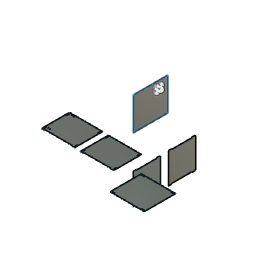
Optical Path Casing (Autodesk Fusion 360 design; units mm, degrees)
Autodesk Fusion 360 part; units mm, degrees
sketch "Sketch2" plane through (0, 0, 0) normal (0, 0, 1) x (1, 0, 0)
  line L0 (32.2949, 19.5332) -> (252.2949, 19.5332)
  line L1 (252.2949, 19.5332) -> (252.2949, -180.4668)
  line L2 (252.2949, -180.4668) -> (32.2949, -180.4668)
  line L3 (32.2949, -180.4668) -> (32.2949, 19.5332)
  line L4 (35.7949, 16.0332) -> (56.7949, 16.0332)
  line L5 (56.7949, 16.0332) -> (56.7949, 12.3332)
  line L6 (56.7949, 12.3332) -> (35.7949, 12.3332)
  line L7 (35.7949, 12.3332) -> (35.7949, 16.0332)
  line L8 (35.7949, -173.2668) -> (56.7949, -173.2668)
  line L9 (56.7949, -173.2668) -> (56.7949, -176.9668)
  line L10 (56.7949, -176.9668) -> (35.7949, -176.9668)
  line L11 (35.7949, -176.9668) -> (35.7949, -173.2668)
  line L12 (227.7949, -173.2668) -> (248.7949, -173.2668)
  line L13 (248.7949, -173.2668) -> (248.7949, -176.9668)
  line L14 (248.7949, -176.9668) -> (227.7949, -176.9668)
  line L15 (227.7949, -176.9668) -> (227.7949, -173.2668)
  line L16 (227.7949, 16.0332) -> (248.7949, 16.0332)
  line L17 (248.7949, 16.0332) -> (248.7949, 12.3332)
  line L18 (248.7949, 12.3332) -> (227.7949, 12.3332)
  line L19 (227.7949, 12.3332) -> (227.7949, 16.0332)
  dimension "d3" = 220
  dimension "d4" = 200
  dimension "d5" = 21
  dimension "d6" = 3.7
  dimension "d7" = 3.5
  dimension "d8" = 3.5
  dimension "d9" = 21
  dimension "d10" = 3.7
  dimension "d11" = 3.5
  dimension "d12" = 3.5
  dimension "d13" = 21
  dimension "d14" = 3.7
  dimension "d15" = 3.5
  dimension "d16" = 3.5
  dimension "d17" = 21
  dimension "d18" = 3.7
  dimension "d19" = 3.5
  dimension "d20" = 3.5
  constraint horizontal L0
  constraint vertical L1
  constraint horizontal L2
  constraint vertical L3
  constraint horizontal L4
  constraint vertical L5
  constraint horizontal L6
  constraint vertical L7
  constraint horizontal L8
  constraint vertical L9
  constraint horizontal L10
  constraint vertical L11
  constraint horizontal L12
  constraint vertical L13
  constraint horizontal L14
  constraint vertical L15
  constraint horizontal L16
  constraint vertical L17
  constraint horizontal L18
  constraint vertical L19
  measures "d3" distance of L0.start L0.end
  measures "d4" distance of L0.start L2.end
  measures "d5" distance of L4.start L4.end
  measures "d6" distance of L4.start L6.end
  measures "d7" distance of L0 L4
  measures "d8" distance of L3 L7
  measures "d9" distance of L8.start L8.end
  measures "d10" distance of L8.start L10.end
  measures "d11" distance of L3 L11
  measures "d12" distance of L2 L10
  measures "d13" distance of L12.start L12.end
  measures "d14" distance of L12.start L14.end
  measures "d15" distance of L2 L14
  measures "d16" distance of L1 L13
  measures "d17" distance of L16.start L16.end
  measures "d18" distance of L16.start L18.end
  measures "d19" distance of L0 L16
  measures "d20" distance of L1 L16.end
sketch "Sketch3" plane through (0, 0, 0) normal (1, 0, 0) x (0, 1, 0)
  line L0 (-1, 5) -> (174, 5)
  line L1 (174, 5) -> (174, -184.5)
  line L2 (174, -184.5) -> (-1, -184.5)
  line L3 (-1, -184.5) -> (-1, 5)
  line L4 (19, 5.0067) -> (-1, 5.0067)
  line L5 (-1, -184.5) -> (19, -184.5)
  line L6 (19, -184.5) -> (19, -188.5)
  line L7 (19, -188.5) -> (-1, -188.5)
  line L8 (-1, -188.5) -> (-1, -184.5)
  line L9 (174, -184.5) -> (164, -184.5)
  line L10 (174, 5) -> (164, 5)
  line L11 (34, -147.5) -> (19, -147.5)
  line L12 (19, -147.5) -> (19, -167.5)
  line L13 (19, -167.5) -> (34, -167.5)
  line L14 (34, -167.5) -> (34, -147.5)
  line L15 (170.5, -184.5) -> (150.5, -184.5)
  line L16 (150.5, -184.5) -> (150.5, -188.5)
  line L17 (150.5, -188.5) -> (170.5, -188.5)
  line L18 (170.5, -188.5) -> (170.5, -184.5)
  line L19 (170.5, 5) -> (150.5, 5)
  line L20 (150.5, 5) -> (150.5, 9)
  line L21 (150.5, 9) -> (170.5, 9)
  line L22 (170.5, 9) -> (170.5, 5)
  line L23 (377.0199, -182.529) -> (377.0199, -186.529)
  line L24 (400.5199, 6.971) -> (400.5199, -182.529)
  line L25 (397.0199, -182.529) -> (377.0199, -182.529)
  line L26 (397.0199, 10.971) -> (397.0199, 6.971)
  line L27 (225.5199, -182.529) -> (225.5199, 6.971)
  line L28 (400.5199, -182.529) -> (380.5199, -182.529)
  line L29 (245.5199, -186.529) -> (225.5199, -186.529)
  line L30 (225.5199, -182.529) -> (245.5199, -182.529)
  line L31 (377.0199, 10.971) -> (397.0199, 10.971)
  line L32 (225.5199, 6.971) -> (400.5199, 6.971)
  line L33 (397.0199, -186.529) -> (397.0199, -182.529)
  line L34 (400.5199, -182.529) -> (225.5199, -182.529)
  line L35 (377.0199, 6.971) -> (377.0199, 10.971)
  line L36 (377.0199, -186.529) -> (397.0199, -186.529)
  line L37 (397.0199, 6.971) -> (377.0199, 6.971)
  line L38 (400.5199, 6.971) -> (380.5199, 6.971)
  line L39 (225.5199, -186.529) -> (225.5199, -182.529)
  line L40 (245.5199, -182.529) -> (245.5199, -186.529)
  line L41 (-1, 5) -> (19, 5)
  line L42 (19, 5) -> (19, 9)
  line L43 (19, 9) -> (-1, 9)
  line L44 (-1, 9) -> (-1, 5)
  line L45 (225.5199, 6.971) -> (245.5199, 6.971)
  line L46 (225.5199, 6.971) -> (245.5199, 6.971)
  line L47 (245.5199, 6.971) -> (245.5199, 10.971)
  line L48 (245.5199, 10.971) -> (225.5199, 10.971)
  line L49 (225.5199, 10.971) -> (225.5199, 6.971)
  point P0 (216.5199, 1.971)
  dimension "d29" = 189.5
  dimension "d30" = 175
  dimension "d33" = 20
  dimension "d34" = 4
  dimension "d39" = 15
  dimension "d40" = 20
  dimension "d41" = 20
  dimension "d42" = 17
  dimension "d103" = 20
  dimension "d104" = 4
  dimension "d105" = 3.5
  dimension "d106" = 20
  dimension "d107" = 4
  dimension "d108" = 3.5
  dimension "d109" = 189.5
  dimension "d110" = 175
  dimension "d113" = 20
  dimension "d114" = 4
  dimension "d119" = 20
  dimension "d120" = 4
  dimension "d121" = 3.5
  dimension "d122" = 20
  dimension "d123" = 4
  dimension "d124" = 3.5
  dimension "d163" = 20
  dimension "d164" = 4
  dimension "d167" = 20
  dimension "d169" = 20
  dimension "d170" = 4
  constraint horizontal L0
  constraint vertical L1
  constraint horizontal L2
  constraint vertical L3
  constraint horizontal L4
  constraint horizontal L5
  constraint vertical L6
  constraint horizontal L7
  constraint vertical L8
  constraint horizontal L9
  constraint horizontal L10
  constraint horizontal L11
  constraint vertical L12
  constraint horizontal L13
  constraint vertical L14
  constraint horizontal L15
  constraint vertical L16
  constraint horizontal L17
  constraint vertical L18
  constraint coincident L2 L15.start
  constraint horizontal L19
  constraint vertical L20
  constraint horizontal L21
  constraint vertical L22
  constraint coincident L10 L19.start
  constraint horizontal L32
  constraint vertical L24
  constraint horizontal L34
  constraint vertical L27
  constraint horizontal L30
  constraint vertical L40
  constraint horizontal L29
  constraint vertical L39
  constraint horizontal L28
  constraint horizontal L38
  constraint horizontal L25
  constraint vertical L23
  constraint horizontal L36
  constraint vertical L33
  constraint coincident L25.start L34
  constraint horizontal L37
  constraint vertical L35
  constraint horizontal L31
  constraint vertical L26
  constraint coincident L26.end L38
  constraint horizontal L41
  constraint vertical L42
  constraint horizontal L43
  constraint vertical L44
  constraint horizontal L45
  constraint horizontal L46
  constraint vertical L47
  constraint horizontal L48
  constraint vertical L49
  measures "d29" distance of L0.start L2.end
  measures "d30" distance of L0.start L0.end
  measures "d33" distance of L2.end L5.end
  measures "d34" distance of L2.end L7.end
  measures "d39" distance of L11.start L11.end
  measures "d40" distance of L11.start L13.end
  measures "d41" distance of L3 L12
  measures "d42" distance of L2 L13
  measures "d103" distance of L15.start L15.end
  measures "d104" distance of L15.start L17.end
  measures "d105" distance of L1 L18
  measures "d106" distance of L19.start L19.end
  measures "d107" distance of L19.start L21.end
  measures "d108" distance of L1 L22
  measures "d109" distance of L27.start L27.end
  measures "d110" distance of L24.start L27.end
  measures "d113" distance of L27.start L30.end
  measures "d114" distance of L27.start L29.end
  measures "d119" distance of L25.start L23.start
  measures "d120" distance of L25.start L33.start
  measures "d121" distance of L24 L33
  measures "d122" distance of L35.start L26.end
  measures "d123" distance of L26.start L26.end
  measures "d124" distance of L24 L26
  measures "d163" distance of L0.start L41.end
  measures "d164" distance of L0.start L43.end
  measures "d167" distance of L27.end L45.end
  measures "d169" distance of L27.end L45.end
  measures "d170" distance of L27.end L48.end
sketch "Sketch5" plane through (0, 0, 0) normal (0, 0, 1) x (1, 0, 0)
  line L0 (-287.8095, 127.6155) -> (-74.8095, 127.6155)
  line L1 (-74.8095, 127.6155) -> (-74.8095, -47.3845)
  line L2 (-74.8095, -47.3845) -> (-287.8095, -47.3845)
  line L3 (-287.8095, -47.3845) -> (-287.8095, 127.6155)
  line L4 (-287.8095, -47.3845) -> (-267.8095, -47.3845)
  line L5 (-267.8095, -47.3845) -> (-267.8095, -50.8845)
  line L6 (-267.8095, -50.8845) -> (-287.8095, -50.8845)
  line L7 (-287.8095, -50.8845) -> (-287.8095, -47.3845)
  line L8 (-74.8095, -47.3845) -> (-94.8095, -47.3845)
  line L9 (-94.8095, -47.3845) -> (-94.8095, -50.8845)
  line L10 (-94.8095, -50.8845) -> (-74.8095, -50.8845)
  line L11 (-74.8095, -50.8845) -> (-74.8095, -47.3845)
  line L12 (-284.3095, -47.3835) -> (-280.6095, -47.3835)
  line L13 (-280.6095, -47.3835) -> (-280.6095, -26.3835)
  line L14 (-280.6095, -26.3835) -> (-284.3095, -26.3835)
  line L15 (-284.3095, -26.3835) -> (-284.3095, -47.3835)
  line L16 (-78.3095, -47.3348) -> (-82.0095, -47.3348)
  line L17 (-82.0095, -47.3348) -> (-82.0095, -26.3348)
  line L18 (-82.0095, -26.3348) -> (-78.3095, -26.3348)
  line L19 (-78.3095, -26.3348) -> (-78.3095, -47.3348)
  line L20 (-326.8625, -44.8366) -> (-539.8625, -44.8366)
  line L21 (-326.8625, -44.8366) -> (-346.8625, -44.8366)
  line L22 (-330.3625, -44.7869) -> (-334.0625, -44.7869)
  line L23 (-326.8625, -48.3366) -> (-326.8625, -44.8366)
  line L24 (-539.8625, 130.1634) -> (-326.8625, 130.1634)
  line L25 (-330.3625, -23.7869) -> (-330.3625, -44.7869)
  line L26 (-346.8625, -48.3366) -> (-326.8625, -48.3366)
  line L27 (-334.0625, -44.7869) -> (-334.0625, -23.7869)
  line L28 (-346.8625, -44.8366) -> (-346.8625, -48.3366)
  line L29 (-334.0625, -23.7869) -> (-330.3625, -23.7869)
  line L30 (-532.6625, -23.8356) -> (-536.3625, -23.8356)
  line L31 (-539.8625, -48.3366) -> (-539.8625, -44.8366)
  line L32 (-536.3625, -44.8356) -> (-532.6625, -44.8356)
  line L33 (-519.8625, -48.3366) -> (-539.8625, -48.3366)
  line L34 (-539.8625, -44.8366) -> (-539.8625, 130.1634)
  line L35 (-519.8625, -44.8366) -> (-519.8625, -48.3366)
  line L36 (-326.8625, 130.1634) -> (-326.8625, -44.8366)
  line L37 (-536.3625, -23.8356) -> (-536.3625, -44.8356)
  line L38 (-532.6625, -44.8356) -> (-532.6625, -23.8356)
  line L39 (-539.8625, -44.8366) -> (-519.8625, -44.8366)
  circle A0 centre (-521, -24.8366) radius 2
  circle A1 centre (-510, -24.8366) radius 2
  line L40 (-536.3625, 126.6634) -> (-532.6625, 126.6634)
  line L41 (-532.6625, 126.6634) -> (-532.6625, 105.6634)
  line L42 (-532.6625, 105.6634) -> (-536.3625, 105.6634)
  line L43 (-536.3625, 105.6634) -> (-536.3625, 126.6634)
  line L44 (-334.0625, 126.6634) -> (-330.3625, 126.6634)
  line L45 (-330.3625, 126.6634) -> (-330.3625, 105.6634)
  line L46 (-330.3625, 105.6634) -> (-334.0625, 105.6634)
  line L47 (-334.0625, 105.6634) -> (-334.0625, 126.6634)
  line L48 (-284.3095, 124.1155) -> (-280.6095, 124.1155)
  line L49 (-280.6095, 124.1155) -> (-280.6095, 103.1155)
  line L50 (-280.6095, 103.1155) -> (-284.3095, 103.1155)
  line L51 (-284.3095, 103.1155) -> (-284.3095, 124.1155)
  line L52 (-82.0095, 124.1155) -> (-78.3095, 124.1155)
  line L53 (-78.3095, 124.1155) -> (-78.3095, 103.1155)
  line L54 (-78.3095, 103.1155) -> (-82.0095, 103.1155)
  line L55 (-82.0095, 103.1155) -> (-82.0095, 124.1155)
  line L56 (-497.8625, 124.1634) -> (-519.8625, 124.1634)
  line L57 (-519.8625, 124.1634) -> (-519.8625, 121.1634)
  line L58 (-519.8625, 121.1634) -> (-497.8625, 121.1634)
  line L59 (-497.8625, 121.1634) -> (-497.8625, 124.1634)
  dimension "d57" = 213
  dimension "d58" = 175
  dimension "d59" = 20
  dimension "d60" = 3.5
  dimension "d61" = 20
  dimension "d62" = 3.5
  dimension "d63" = 3.7
  dimension "d64" = 21
  dimension "d65" = 0.001
  dimension "d66" = 3.5
  dimension "d67" = 3.7
  dimension "d68" = 21
  dimension "d69" = 3.5
  dimension "d70" = 213
  dimension "d71" = 175
  dimension "d72" = 20
  dimension "d73" = 3.5
  dimension "d74" = 20
  dimension "d75" = 3.5
  dimension "d76" = 3.7
  dimension "d77" = 21
  dimension "d78" = 0.001
  dimension "d79" = 3.5
  dimension "d80" = 3.7
  dimension "d81" = 21
  dimension "d82" = 3.5
  dimension "d83" = 4
  dimension "d84" = 4
  dimension "d85" = 11
  dimension "d86" = 20
  dimension "d87" = 3.7
  dimension "d88" = 21
  dimension "d89" = 3.5
  dimension "d90" = 3.5
  dimension "d91" = 3.7
  dimension "d92" = 21
  dimension "d93" = 3.5
  dimension "d94" = 3.5
  dimension "d95" = 3.7
  dimension "d96" = 21
  dimension "d97" = 3.5
  dimension "d98" = 3.5
  dimension "d99" = 3.7
  dimension "d100" = 21
  dimension "d101" = 3.5
  dimension "d102" = 3.5
  dimension "d125" = 22
  dimension "d126" = 3
  dimension "d127" = 6
  dimension "d128" = 20
  constraint horizontal L0
  constraint vertical L1
  constraint horizontal L2
  constraint vertical L3
  constraint horizontal L4
  constraint vertical L5
  constraint horizontal L6
  constraint vertical L7
  constraint horizontal L8
  constraint vertical L9
  constraint horizontal L10
  constraint vertical L11
  constraint horizontal L12
  constraint vertical L13
  constraint horizontal L14
  constraint vertical L15
  constraint horizontal L16
  constraint vertical L17
  constraint horizontal L18
  constraint vertical L19
  constraint horizontal L24
  constraint vertical L36
  constraint horizontal L20
  constraint vertical L34
  constraint horizontal L39
  constraint vertical L35
  constraint horizontal L33
  constraint vertical L31
  constraint horizontal L21
  constraint vertical L28
  constraint horizontal L26
  constraint vertical L23
  constraint horizontal L32
  constraint vertical L38
  constraint horizontal L30
  constraint vertical L37
  constraint horizontal L22
  constraint vertical L27
  constraint horizontal L29
  constraint vertical L25
  constraint horizontal L40
  constraint vertical L41
  constraint horizontal L42
  constraint vertical L43
  constraint horizontal L44
  constraint vertical L45
  constraint horizontal L46
  constraint vertical L47
  constraint horizontal L48
  constraint vertical L49
  constraint horizontal L50
  constraint vertical L51
  constraint horizontal L52
  constraint vertical L53
  constraint horizontal L54
  constraint vertical L55
  constraint horizontal L56
  constraint vertical L57
  constraint horizontal L58
  constraint vertical L59
  measures "d57" distance of L0.start L0.end
  measures "d58" distance of L0.start L2.end
  measures "d59" distance of L2.end L4.end
  measures "d60" distance of L2.end L6.end
  measures "d61" distance of L1.end L8.end
  measures "d62" distance of L1.end L10.end
  measures "d63" distance of L12.start L12.end
  measures "d64" distance of L12.start L14.end
  measures "d65" distance of L2 L12
  measures "d66" distance of L3 L15
  measures "d67" distance of L16.start L16.end
  measures "d68" distance of L16.start L18.end
  measures "d69" distance of L1 L19
  measures "d70" distance of L24.end L24.start
  measures "d71" distance of L20.end L24.start
  measures "d72" distance of L20.end L35.start
  measures "d73" distance of L20.end L31.start
  measures "d74" distance of L20.start L21.end
  measures "d75" distance of L20.start L23.start
  measures "d76" distance of L32.start L32.end
  measures "d77" distance of L32.start L30.end
  measures "d78" distance of L20 L32
  measures "d79" distance of L34 L37
  measures "d80" distance of L22.end L22.start
  measures "d81" distance of L22.start L25.start
  measures "d82" distance of L25 L36
  measures "d83" diameter of A0
  measures "d84" diameter of A1
  measures "d85" distance of A0.centre A1.centre
  measures "d86" distance of L20 A0.centre
  measures "d87" distance of L40.start L40.end
  measures "d88" distance of L40.start L42.end
  measures "d89" distance of L34 L43
  measures "d90" distance of L24 L40
  measures "d91" distance of L44.start L44.end
  measures "d92" distance of L44.start L46.end
  measures "d93" distance of L36 L45
  measures "d94" distance of L24 L44.start
  measures "d95" distance of L48.start L48.end
  measures "d96" distance of L48.start L50.end
  measures "d97" distance of L0 L48
  measures "d98" distance of L3 L51
  measures "d99" distance of L52.start L52.end
  measures "d100" distance of L52.start L54.end
  measures "d101" distance of L1 L53
  measures "d102" distance of L0 L52
  measures "d125" distance of L56.start L56.end
  measures "d126" distance of L56 L58
  measures "d127" distance of L24 L56
  measures "d128" distance of L34 L57
extrude "Extrude1" add sketch "Sketch5" along normal blind 1 contours L20 L21 L24 L34 L36 L39 makes body 1
extrude "Extrude2" add sketch "Sketch5" along normal blind 1 contours L20 L31 L33 L35 L39 bodies 1
extrude "Extrude3" add sketch "Sketch5" along normal blind 1 contours L20 L21 L23 L26 L28 bodies 1
extrude "Extrude4" add sketch "Sketch5" along normal blind 1 separate body contours L0 L1 L2 L3 L4 L8 makes body 2
extrude "Extrude5" add sketch "Sketch5" along normal blind 1 contours L2 L4 L5 L6 L7 bodies 2
extrude "Extrude6" add sketch "Sketch5" along normal blind 1 contours L2 L8 L9 L10 L11 bodies 2
extrude "Extrude7" add sketch "Sketch2" along normal blind 1 separate body makes body 3
extrude "Extrude8" add sketch "Sketch3" along normal blind 1 separate body contours L24 L25 L27 L28 L30 L32 L34 L37 L38 L45 L46 makes body 4
extrude "Extrude9" add sketch "Sketch3" along normal blind 1 contours L29 L30 L34 L39 L40 bodies 4
extrude "Extrude10" add sketch "Sketch3" along normal blind 1 contours L23 L25 L28 L33 L34 L36 bodies 4
extrude "Extrude11" add sketch "Sketch3" along normal blind 1 separate body contours L0 L1 L2 L3 L5 L9 L10 L15 L19 L41 makes body 5
extrude "Extrude12" add sketch "Sketch3" along normal blind 1 contours L2 L9 L15 L16 L17 L18 bodies 5
extrude "Extrude13" add sketch "Sketch3" along normal blind 1 contours L2 L5 L6 L7 L8 bodies 5
extrude "Extrude14" add sketch "Sketch3" along normal blind 1 separate body contours L0 L4 L41 L42 L44 | L4 L42 L43 L44 makes body 6
extrude "Extrude15" add sketch "Sketch3" along normal blind 1 contours L0 L10 L19 L20 L21 L22 bodies 5
extrude "Extrude17" add sketch "Sketch3" along normal blind 1 contours L26 L31 L32 L35 L37 L38 bodies 4
combine "Combine1" operation add target body 5 tool bodies 6
extrude "Extrude18" add sketch "Sketch3" along normal blind 1 contours L32 L45 L46 L47 L48 L49 bodies 4
sketch "Side 2" plane through (0, 0, 1) normal (0, 0, 1) x (-1, 0, 0)
  line L0 (497.8625, -124.1634) -> (497.8625, -121.1634)
  line L1 (497.8625, -121.1634) -> (519.8625, -121.1634)
  line L2 (519.8625, -121.1634) -> (519.8625, -124.1634)
  line L3 (519.8625, -124.1634) -> (497.8625, -124.1634)
  line L4 (330.3625, -105.6634) -> (334.0625, -105.6634)
  line L5 (334.0625, -105.6634) -> (334.0625, -126.6634)
  line L6 (334.0625, -126.6634) -> (330.3625, -126.6634)
  line L7 (330.3625, -126.6634) -> (330.3625, -105.6634)
  circle A0 centre (521, 24.8366) radius 2
  circle A1 centre (510, 24.8366) radius 2
  line L8 (532.6625, -105.6634) -> (536.3625, -105.6634)
  line L9 (536.3625, -105.6634) -> (536.3625, -126.6634)
  line L10 (536.3625, -126.6634) -> (532.6625, -126.6634)
  line L11 (532.6625, -126.6634) -> (532.6625, -105.6634)
  line L12 (532.6625, 23.8356) -> (532.6625, 44.8356)
  line L13 (532.6625, 44.8356) -> (536.3625, 44.8356)
  line L14 (536.3625, 44.8356) -> (536.3625, 23.8356)
  line L15 (536.3625, 23.8356) -> (532.6625, 23.8356)
  line L16 (334.0625, 44.7869) -> (334.0625, 23.7869)
  line L17 (334.0625, 23.7869) -> (330.3625, 23.7869)
  line L18 (330.3625, 23.7869) -> (330.3625, 44.7869)
  line L19 (330.3625, 44.7869) -> (334.0625, 44.7869)
  line L20 (539.8625, -130.1634) -> (539.8625, 48.3366)
  line L21 (539.8625, 48.3366) -> (519.8625, 48.3366)
  line L22 (519.8625, 48.3366) -> (519.8625, 44.8366)
  line L23 (519.8625, 44.8366) -> (346.8625, 44.8366)
  line L24 (346.8625, 44.8366) -> (346.8625, 48.3366)
  line L25 (346.8625, 48.3366) -> (326.8625, 48.3366)
  line L26 (326.8625, 48.3366) -> (326.8625, -130.1634)
  line L27 (326.8625, -130.1634) -> (539.8625, -130.1634)
sketch "Side 3" plane through (0, 0, 1) normal (0, 0, 1) x (-1, 0, 0)
  line L0 (280.6095, -103.1155) -> (284.3095, -103.1155)
  line L1 (284.3095, -103.1155) -> (284.3095, -124.1155)
  line L2 (284.3095, -124.1155) -> (280.6095, -124.1155)
  line L3 (280.6095, -124.1155) -> (280.6095, -103.1155)
  line L4 (78.3095, -103.1155) -> (82.0095, -103.1155)
  line L5 (82.0095, -103.1155) -> (82.0095, -124.1155)
  line L6 (82.0095, -124.1155) -> (78.3095, -124.1155)
  line L7 (78.3095, -124.1155) -> (78.3095, -103.1155)
  line L8 (284.3095, 47.3835) -> (284.3095, 26.3835)
  line L9 (284.3095, 26.3835) -> (280.6095, 26.3835)
  line L10 (280.6095, 26.3835) -> (280.6095, 47.3835)
  line L11 (280.6095, 47.3835) -> (284.3095, 47.3835)
  line L12 (82.0095, 26.3348) -> (78.3095, 26.3348)
  line L13 (78.3095, 26.3348) -> (78.3095, 47.3348)
  line L14 (78.3095, 47.3348) -> (82.0095, 47.3348)
  line L15 (82.0095, 47.3348) -> (82.0095, 26.3348)
  line L16 (267.8095, 47.3845) -> (94.8095, 47.3845)
  line L17 (94.8095, 47.3845) -> (94.8095, 50.8845)
  line L18 (94.8095, 50.8845) -> (74.8095, 50.8845)
  line L19 (74.8095, 50.8845) -> (74.8095, -127.6155)
  line L20 (74.8095, -127.6155) -> (287.8095, -127.6155)
  line L21 (287.8095, -127.6155) -> (287.8095, 50.8845)
  line L22 (287.8095, 50.8845) -> (267.8095, 50.8845)
  line L23 (267.8095, 50.8845) -> (267.8095, 47.3845)
sketch "Bottom" plane through (0, 0, 1) normal (0, 0, 1) x (-1, 0, 0)
  line L0 (-56.7949, 176.9668) -> (-35.7949, 176.9668)
  line L1 (-35.7949, 176.9668) -> (-35.7949, 173.2668)
  line L2 (-35.7949, 173.2668) -> (-56.7949, 173.2668)
  line L3 (-56.7949, 173.2668) -> (-56.7949, 176.9668)
  line L4 (-248.7949, 176.9668) -> (-227.7949, 176.9668)
  line L5 (-227.7949, 176.9668) -> (-227.7949, 173.2668)
  line L6 (-227.7949, 173.2668) -> (-248.7949, 173.2668)
  line L7 (-248.7949, 173.2668) -> (-248.7949, 176.9668)
  line L8 (-248.7949, -12.3332) -> (-227.7949, -12.3332)
  line L9 (-227.7949, -12.3332) -> (-227.7949, -16.0332)
  line L10 (-227.7949, -16.0332) -> (-248.7949, -16.0332)
  line L11 (-248.7949, -16.0332) -> (-248.7949, -12.3332)
  line L12 (-56.7949, -12.3332) -> (-35.7949, -12.3332)
  line L13 (-35.7949, -12.3332) -> (-35.7949, -16.0332)
  line L14 (-35.7949, -16.0332) -> (-56.7949, -16.0332)
  line L15 (-56.7949, -16.0332) -> (-56.7949, -12.3332)
  line L16 (-32.2949, 180.4668) -> (-252.2949, 180.4668)
  line L17 (-252.2949, 180.4668) -> (-252.2949, -19.5332)
  line L18 (-252.2949, -19.5332) -> (-32.2949, -19.5332)
  line L19 (-32.2949, -19.5332) -> (-32.2949, 180.4668)
sketch "Side 1" plane through (1, 0, 0) normal (1, 0, 0) x (0, 1, 0)
  line L0 (34, -147.5) -> (34, -167.5)
  line L1 (34, -167.5) -> (19, -167.5)
  line L2 (19, -167.5) -> (19, -147.5)
  line L3 (19, -147.5) -> (34, -147.5)
  line L4 (174, 5) -> (170.5, 5)
  line L5 (170.5, 5) -> (170.5, 9)
  line L6 (170.5, 9) -> (150.5, 9)
  line L7 (150.5, 9) -> (150.5, 5)
  line L8 (150.5, 5) -> (19, 5)
  line L9 (19, 5) -> (19, 9)
  line L10 (19, 9) -> (-1, 9)
  line L11 (-1, 9) -> (-1, -188.5)
  line L12 (-1, -188.5) -> (19, -188.5)
  line L13 (19, -188.5) -> (19, -184.5)
  line L14 (19, -184.5) -> (150.5, -184.5)
  line L15 (150.5, -184.5) -> (150.5, -188.5)
  line L16 (150.5, -188.5) -> (170.5, -188.5)
  line L17 (170.5, -188.5) -> (170.5, -184.5)
  line L18 (170.5, -184.5) -> (174, -184.5)
  line L19 (174, -184.5) -> (174, 5)
sketch "Side 4" plane through (0, 0, 0) normal (-1, 0, 0) x (0, -1, 0)
  line L0 (-400.5199, 6.971) -> (-400.5199, -182.529)
  line L1 (-400.5199, -182.529) -> (-397.0199, -182.529)
  line L2 (-397.0199, -182.529) -> (-397.0199, -186.529)
  line L3 (-397.0199, -186.529) -> (-377.0199, -186.529)
  line L4 (-377.0199, -186.529) -> (-377.0199, -182.529)
  line L5 (-377.0199, -182.529) -> (-245.5199, -182.529)
  line L6 (-245.5199, -182.529) -> (-245.5199, -186.529)
  line L7 (-245.5199, -186.529) -> (-225.5199, -186.529)
  line L8 (-225.5199, -186.529) -> (-225.5199, 10.971)
  line L9 (-225.5199, 10.971) -> (-245.5199, 10.971)
  line L10 (-245.5199, 10.971) -> (-245.5199, 6.971)
  line L11 (-245.5199, 6.971) -> (-377.0199, 6.971)
  line L12 (-377.0199, 6.971) -> (-377.0199, 10.971)
  line L13 (-377.0199, 10.971) -> (-397.0199, 10.971)
  line L14 (-397.0199, 10.971) -> (-397.0199, 6.971)
  line L15 (-397.0199, 6.971) -> (-400.5199, 6.971)
sketch "Top" plane through (0, 0, 0) normal (1, 0, 0) x (0, 1, 0)
  line L0 (0.5748, 432.3565) -> (220.5748, 432.3565)
  line L1 (220.5748, 432.3565) -> (220.5748, 222.3565)
  line L2 (220.5748, 222.3565) -> (0.5748, 222.3565)
  line L3 (0.5748, 222.3565) -> (0.5748, 432.3565)
  circle A0 centre (150, 400) radius 1.05
  circle A1 centre (175, 400) radius 1.05
  circle A2 centre (150, 375) radius 1.05
  circle A3 centre (175, 375) radius 1.05
  dimension "d173" = 220
  dimension "d174" = 210
  dimension "d175" = 2.1
  dimension "d176" = 2.1
  dimension "d177" = 2.1
  dimension "d178" = 2.1
  constraint horizontal L0
  constraint vertical L1
  constraint horizontal L2
  constraint vertical L3
  measures "d173" distance of L0.start L0.end
  measures "d174" distance of L0.start L2.end
  measures "d175" diameter of A0
  measures "d176" diameter of A1
  measures "d177" diameter of A2
  measures "d178" diameter of A3
extrude "Extrude19" add sketch "Top" along normal blind 1 separate body makes body 7
sketch "Sketch13" plane through (1, 0, 0) normal (1, 0, 0) x (0, 1, 0)
